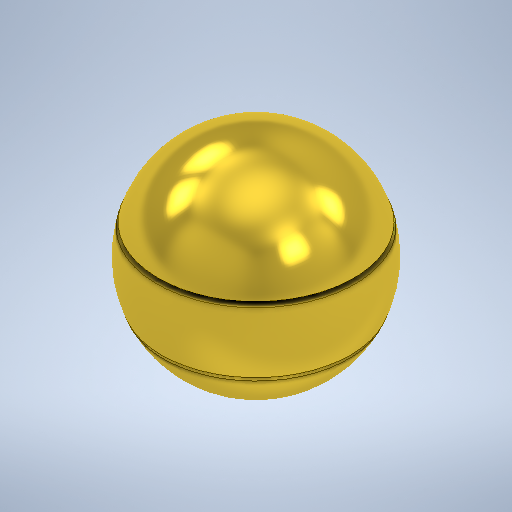
# Autodesk Inventor part: Sessao8_07_04_2025_0003_0001
Saved by Autodesk Inventor 2025.2 (Build 292293000, 293)
## iProperties
Created: 2025-04-07
Part Number: Sessao8_07_04_2025_0003_0001
Material: Ouro
Document SubType Name: Modeling
Designer: Gustavo Sousa
Density: 19.3 g/cm^3
Appearance: Metal quente 2400F
Author: Gustavo Sousa
Autodesk Inventor part; units mm, degrees
ref_plane "YZ Plane" through (0, 0, 0) normal (1, 0, 0) x (0, 1, 0)
ref_plane "XZ Plane" through (0, 0, 0) normal (0, 1, 0) x (-1, 0, 0)
ref_plane "XY Plane" through (0, 0, 0) normal (0, 0, 1) x (1, 0, 0)
sketch "Esboço1" plane through (0, 0, 0) normal (0, 0, 1) x (1, 0, 0)
  circle A0 centre (0, 0) radius 10 construction
  arc A1 (0, 10) -> (0, -10) centre (0, 0) ccw
  line L0 (0, 10) -> (0, 0)
  line L1 (0, 0) -> (0, -10)
  line L2 (-14, 0) -> (14, 0) projected
  line L3 (0, -38.2) -> (0, 36.7) projected
  line L4 (0, 0) -> (0, -2) construction
  arc A2 (9.259, -3.7778) -> (-9.259, -3.7778) centre (0, -27) ccw
  line L5 (0, 2) -> (0, 0) construction
  arc A3 (-9.5691, 2.9038) -> (9.5691, 2.9038) centre (0, 26) ccw
  arc A4 (9.0731, -4.2045) -> (-9.0731, -4.2045) centre (0, -27.5) ccw
  arc A5 (-9.6937, 2.4559) -> (9.6937, 2.4559) centre (0, 25.5) ccw
  point P0 (0, 1)
  point P1 (0, -2.5)
  point P2 (0, 0.5)
  point P3 (0, -2.5)
  point P4 (0, -2)
  point P5 (0, 0.5)
  point P6 (0, 1)
  dimension "d0" = 20
  dimension "d6" = 2
  dimension "d7" = 25
  dimension "d8" = 0.5
  dimension "d9" = 0.5
  constraints: 24 point on circle, 8 end point, 6 centre point, 5 vertical alignment, 3 equal radius, 2 collinear, 2 vertical, 1 coincident, 1 concentric, 1 midpoint, 1 point on line
  measures "d0" diameter of A0
  measures "d6" distance of L4.end L0.end
  measures "d7" radius of A2
  measures "d8" distance of A2.centre A4.centre
  measures "d9" distance of A3.centre A5.centre
revolve "Revolução1" add sketch "Esboço1" angle 360 mid plane about axis through (0, -10, 0) along (0, 1, 0)
revolve "Revolução2" cut sketch "Esboço1" angle 360 about axis through (0, -10, 0) along (0, 1, 0) contours A3 L0 A5 A1 | A2 L1 A4 A1
